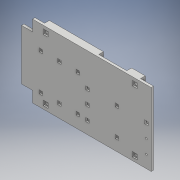
# Autodesk Inventor part: foot_printed
Saved by Autodesk Inventor 2018 (Build 220112000, 112)
## iProperties
Created: 2020-01-31
Part Number: foot_printed
Material: Generic
Document SubType Name: Modeling
Designer: bitbots
Density: 1 g/cm^3
Appearance: Default
Author: bitbots
Autodesk Inventor part; units mm, degrees
ref_plane "YZ Plane" through (0, 0, 0) normal (1, 0, 0) x (0, 1, 0)
ref_plane "XZ Plane" through (0, 0, 0) normal (0, 1, 0) x (-1, 0, 0)
ref_plane "XY Plane" through (0, 0, 0) normal (0, 0, 1) x (1, 0, 0)
sketch "Sketch1" plane through (0, 0, 0) normal (0, 1, 0) x (-1, 0, 0)
  line L0 (-65, 45) -> (65, 45) construction
  line L1 (65, 45) -> (65, -45) construction
  line L2 (65, -45) -> (-65, -45) construction
  line L3 (-65, -45) -> (-65, 45) construction
  line L4 (-65, 45) -> (65, -45) construction
  line L5 (65, 45) -> (-65, -45) construction
  circle A0 centre (65, 45) radius 2.1
  circle A1 centre (65, -45) radius 2.1
  circle A2 centre (-65, -45) radius 2.1
  circle A3 centre (-65, 45) radius 2.1
  line L6 (65, 45) -> (65, 19) construction
  line L7 (65, 19) -> (72, 19) construction
  line L8 (72, 19) -> (72, -34) construction
  line L9 (72, -34) -> (18, -34) construction
  line L10 (18, -34) -> (18, 19) construction
  line L11 (18, 19) -> (45, 19) construction
  line L12 (18, -34) -> (45, -34) construction
  circle A4 centre (45, -34) radius 1.35
  circle A5 centre (18, -34) radius 1.35
  circle A6 centre (18, 19) radius 1.35
  circle A7 centre (45, 19) radius 1.35
  circle A8 centre (72, -34) radius 1.35
  circle A9 centre (72, 19) radius 1.35
  line L13 (-65, -45) -> (-65, -35) construction
  line L14 (-65, -35) -> (-82, -35) construction
  circle A10 centre (-82, -35) radius 1.35
  line L15 (-82, -35) -> (-39, -35) construction
  line L16 (-39, -35) -> (4, -35) construction
  line L17 (4, -35) -> (4, -15) construction
  line L18 (4, -15) -> (4, 5) construction
  line L19 (4, 5) -> (-39, 5) construction
  line L20 (-39, 5) -> (-82, 5) construction
  circle A11 centre (-39, -35) radius 1.35
  circle A12 centre (4, -35) radius 1.35
  circle A13 centre (4, -15) radius 1.35
  circle A14 centre (4, 5) radius 1.35
  circle A15 centre (-39, 5) radius 1.35
  circle A16 centre (-82, 5) radius 1.35
  line L21 (-65, -45) -> (-65, -53) construction
  line L22 (-65, 45) -> (-65, 53) construction
  line L23 (65, -45) -> (65, -53) construction
  line L24 (65, 45) -> (70, 45) construction
  line L25 (65, 45) -> (65, 53) construction
  line L26 (-65, 45) -> (-70, 45) construction
  line L27 (-82, -35) -> (-89, -35) construction
  line L28 (-89, -35) -> (-89, -53)
  line L29 (-65, -53) -> (-89, -53)
  line L30 (-65, 53) -> (-89, 53)
  line L31 (-89, 53) -> (-89, -35)
  line L32 (-65, -53) -> (65, -53)
  line L33 (-65, 53) -> (65, 53)
  line L34 (65, -45) -> (100, -45) construction
  line L35 (100, -45) -> (100, -53)
  line L36 (100, -53) -> (65, -53)
  line L37 (65, 53) -> (100, 53)
  line L38 (100, 53) -> (100, -45)
  line L39 (-82, 5) -> (-82, -15) construction
  circle A17 centre (-82, -15) radius 1.35
  point P0 (0, 0)
  dimension "d0" = 130
  dimension "d1" = 90
  dimension "d2" = 4.2
  dimension "d3" = 4.2
  dimension "d4" = 4.2
  dimension "d5" = 4.2
  dimension "d6" = 26
  dimension "d7" = 7
  dimension "d8" = 53
  dimension "d9" = 54
  dimension "d10" = 53
  dimension "d11" = 27
  dimension "d12" = 27
  dimension "d13" = 2.7
  dimension "d14" = 2.7
  dimension "d15" = 2.7
  dimension "d16" = 2.7
  dimension "d17" = 2.7
  dimension "d18" = 2.7
  dimension "d19" = 10
  dimension "d20" = 17
  dimension "d21" = 2.7
  dimension "d22" = 43
  dimension "d23" = 43
  dimension "d24" = 20
  dimension "d26" = 20
  dimension "d27" = 43
  dimension "d28" = 43
  dimension "d29" = 2.7
  dimension "d30" = 2.7
  dimension "d31" = 2.7
  dimension "d32" = 2.7
  dimension "d33" = 2.7
  dimension "d34" = 2.7
  dimension "d35" = 8
  dimension "d36" = 8
  dimension "d38" = 8
  dimension "d40" = 5
  dimension "d41" = 8
  dimension "d42" = 5
  dimension "d43" = 7
  dimension "d44" = 35
  dimension "d54" = 20
  dimension "d55" = 2.7
  constraints: 80 end point, 18 centre point, 18 coincident, 14 perpendicular, 7 horizontal, 6 point on line, 6 vertical, 3 midpoint, 3 parallel
  measures "d0" distance of L1.end L2.end
  measures "d1" distance of L0.end L1.end
  measures "d2" diameter of A0
  measures "d3" diameter of A1
  measures "d4" diameter of A2
  measures "d5" diameter of A3
  measures "d6" distance of L6.start L6.end
  measures "d7" distance of L6.end L7.end
  measures "d8" distance of L7.end L8.end
  measures "d9" distance of L8.end L9.end
  measures "d10" distance of L9.end L10.end
  measures "d11" distance of L10.end L11.end
  measures "d12" distance of L9.end L12.end
  measures "d13" diameter of A4
  measures "d14" diameter of A5
  measures "d15" diameter of A6
  measures "d16" diameter of A7
  measures "d17" diameter of A8
  measures "d18" diameter of A9
  measures "d19" distance of L13.start L13.end
  measures "d20" distance of L13.end L14.end
  measures "d21" diameter of A10
  measures "d22" distance of L15.start L15.end
  measures "d23" distance of L15.end L16.end
  measures "d24" distance of L16.end L17.end
  measures "d26" distance of L17.end L18.end
  measures "d27" distance of L18.end L19.end
  measures "d28" distance of L19.end L20.end
  measures "d29" diameter of A11
  measures "d30" diameter of A12
  measures "d31" diameter of A13
  measures "d32" diameter of A14
  measures "d33" diameter of A15
  measures "d34" diameter of A16
  measures "d35" distance of L13.start L21.end
  measures "d36" distance of L22.start L22.end
  measures "d38" distance of L23.start L23.end
  measures "d40" distance of L6.start L24.end
  measures "d41" distance of L6.start L25.end
  measures "d42" distance of L22.start L26.end
  measures "d43" distance of L15.start L27.end
  measures "d44" distance of L23.start L34.end
  measures "d54" distance of L39.start L39.end
  measures "d55" diameter of A17
extrude "Extrusion1" add sketch "Sketch1" along normal blind 3.5
sketch "Sketch2" plane through (0, 3.5, 0) normal (0, 1, 0) x (1, 0, 0)
  circle A0 centre (65, -45) radius 2.1 construction
  circle A1 centre (65, 45) radius 2.1 construction
  circle A2 centre (-65, 45) radius 2.1 construction
  circle A3 centre (-65, -45) radius 2.1 construction
  circle A4 centre (82, -5) radius 1.35 construction
  circle A5 centre (39, -5) radius 1.35 construction
  circle A6 centre (-4, -5) radius 1.35 construction
  circle A7 centre (-4, 15) radius 1.35 construction
  circle A8 centre (-4, 35) radius 1.35 construction
  circle A9 centre (39, 35) radius 1.35 construction
  circle A10 centre (82, 35) radius 1.35 construction
  circle A11 centre (-72, -19) radius 1.35 construction
  circle A12 centre (-72, 34) radius 1.35 construction
  circle A13 centre (-45, -19) radius 1.35 construction
  circle A14 centre (-18, -19) radius 1.35 construction
  circle A15 centre (-18, 34) radius 1.35 construction
  circle A16 centre (-45, 34) radius 1.35 construction
  line L0 (89, 53) -> (-100, 53) construction
  line L1 (-100, 53) -> (-100, -53) construction
  line L2 (-100, -53) -> (89, -53) construction
  line L3 (89, -53) -> (89, 53) construction
  line L4 (65, -45) -> (65, -49.25) construction
  line L5 (65, -49.25) -> (60.75, -49.25)
  line L6 (60.75, -49.25) -> (60.75, -40.75)
  line L7 (60.75, -40.75) -> (65, -40.75)
  line L8 (65, -49.25) -> (70, -49.25)
  line L9 (65, -40.75) -> (70, -40.75)
  line L10 (89, -53) -> (-100, -53) construction
  line L11 (89, -53) -> (89, 53) construction
  line L12 (89, 0) -> (-100, 0) construction
  line L13 (0, 0) -> (0, 53) construction
  line L14 (89, 53) -> (-100, 53) construction
  line L15 (0, 0) -> (0, -53) construction
  line L16 (65, 49.25) -> (60.75, 49.25)
  line L17 (60.75, 49.25) -> (60.75, 40.75)
  line L18 (60.75, 40.75) -> (65, 40.75)
  line L19 (65, 49.25) -> (70, 49.25)
  line L20 (65, 40.75) -> (70, 40.75)
  line L21 (-65, -49.25) -> (-60.75, -49.25)
  line L22 (-60.75, -49.25) -> (-60.75, -40.75)
  line L23 (-60.75, -40.75) -> (-65, -40.75)
  line L24 (-65, -49.25) -> (-70, -49.25)
  line L25 (-65, -40.75) -> (-70, -40.75)
  line L26 (-60.75, 40.75) -> (-65, 40.75)
  line L27 (-65, 40.75) -> (-70, 40.75)
  line L28 (-65, 49.25) -> (-60.75, 49.25)
  line L29 (-65, 49.25) -> (-70, 49.25)
  line L30 (-60.75, 49.25) -> (-60.75, 40.75)
  line L31 (-70, -49.25) -> (-70, -53)
  line L32 (-70, -53) -> (70, -53) construction
  line L33 (70, -53) -> (70, -49.25)
  line L34 (70, 49.25) -> (70, 53)
  line L35 (70, 53) -> (-70, 53)
  line L36 (-70, 53) -> (-70, 49.25)
  line L37 (-70, -40.75) -> (-70, -37)
  circle A17 centre (-4, 35) radius 1.35 construction
  line L38 (-4, 35) -> (-11, 35) construction
  line L39 (-70, 40.75) -> (-70, 37)
  line L40 (-11, 35) -> (-11, 37)
  line L41 (-11, 37) -> (-70, 37)
  line L42 (-11, 35) -> (-11, -37)
  line L43 (-11, -37) -> (-70, -37)
  line L44 (-11, -37) -> (9, -37) construction
  line L45 (9, -37) -> (9, -53)
  line L46 (-100, -53) -> (89, -53) construction
  circle A18 centre (39, -5) radius 1.35 construction
  line L47 (39, -5) -> (39, -9) construction
  line L48 (39, -9) -> (9, -9) construction
  line L49 (9, -9) -> (9, -37)
  line L50 (9, -9) -> (-11, -9)
  line L51 (-4, 35) -> (-4, 39) construction
  line L52 (-4, 39) -> (-11, 39)
  line L53 (-11, 39) -> (-11, 37)
  line L54 (-4, 39) -> (70, 39)
  line L55 (70, 39) -> (70, 40.75)
  line L56 (70, -40.75) -> (70, -9)
  line L57 (-70, -53) -> (9, -53)
  line L58 (70, -53) -> (50, -53)
  line L59 (50, -53) -> (50, -9)
  line L60 (50, -9) -> (70, -9)
  dimension "d47" = 4.25
  dimension "d49" = 4.25
  dimension "d50" = 8.5
  dimension "d51" = 5
  dimension "d52" = 5
  dimension "d53" = 3.75
  dimension "d56" = 7
  dimension "d57" = 3.75
  dimension "d58" = 20
  dimension "d59" = 4
  dimension "d60" = 4
  dimension "d62" = 20
  constraints: 106 end point, 18 symmetric about line, 15 perpendicular, 12 point on line, 8 horizontal, 8 vertical, 2 midpoint, 1 collinear
  measures "d47" distance of L4.start L4.end
  measures "d49" distance of L4.end L5.end
  measures "d50" distance of L5.end L6.end
  measures "d51" distance of L4.end L8.end
  measures "d52" distance of L7.end L9.end
  measures "d53" distance of L25.end L37.end
  measures "d56" distance of L38.start L38.end
  measures "d57" distance of L27.end L39.end
  measures "d58" distance of L42.end L44.end
  measures "d59" distance of L47.start L47.end
  measures "d60" distance of L38.start L51.end
  measures "d62" distance of L32.end L58.end
extrude "Extrusion2" add sketch "Sketch2" along normal blind 7
sketch "Sketch3" plane through (0, 3.5, 0) normal (0, 1, 0) x (1, 0, 0)
  circle A0 centre (-45, 34) radius 1.35 construction
  circle A1 centre (-18, 34) radius 1.35 construction
  circle A2 centre (-18, -19) radius 1.35 construction
  circle A3 centre (-45, -19) radius 1.35 construction
  circle A4 centre (-72, 34) radius 1.35 construction
  circle A5 centre (-72, -19) radius 1.35 construction
  circle A6 centre (82, 35) radius 1.35 construction
  circle A7 centre (39, 35) radius 1.35 construction
  circle A8 centre (-4, 35) radius 1.35 construction
  circle A9 centre (-4, 15) radius 1.35 construction
  circle A10 centre (-4, -5) radius 1.35 construction
  circle A11 centre (39, -5) radius 1.35 construction
  circle A12 centre (82, -5) radius 1.35 construction
  circle A13 centre (82, 15) radius 1.35 construction
  circle A14 centre (-65, -45) radius 2.1 projected
  circle A15 centre (-65, 45) radius 2.1 projected
  circle A16 centre (65, 45) radius 2.1 projected
  circle A17 centre (65, -45) radius 2.1 projected
  line L0 (-70, -53) -> (-70, -49.25) projected
  line L1 (-70, -49.25) -> (-60.75, -49.25) projected
  line L2 (-60.75, -49.25) -> (-60.75, -40.75) projected
  line L3 (-60.75, -40.75) -> (-70, -40.75) projected
  line L4 (-70, -40.75) -> (-70, -37) projected
  line L5 (-70, -37) -> (-11, -37) construction
  line L6 (-11, -37) -> (-11, -9) construction
  line L7 (-11, -9) -> (9, -9) construction
  line L8 (9, -9) -> (9, -53) construction
  line L9 (9, -53) -> (50, -53) construction
  line L10 (50, -53) -> (50, -9) construction
  line L11 (50, -9) -> (70, -9) construction
  line L12 (70, -9) -> (70, -40.75) construction
  line L13 (70, -40.75) -> (60.75, -40.75) projected
  line L14 (60.75, -40.75) -> (60.75, -49.25) projected
  line L15 (60.75, -49.25) -> (70, -49.25) projected
  line L16 (70, -49.25) -> (70, -53) construction
  line L17 (70, -53) -> (89, -53) construction
  line L18 (89, -53) -> (89, 53) construction
  line L19 (89, 53) -> (70, 53) construction
  line L20 (70, 53) -> (70, 49.25) projected
  line L21 (70, 49.25) -> (60.75, 49.25) projected
  line L22 (60.75, 49.25) -> (60.75, 40.75) projected
  line L23 (60.75, 40.75) -> (70, 40.75) projected
  line L24 (70, 40.75) -> (70, 39) projected
  line L25 (70, 39) -> (-11, 39) construction
  line L26 (-11, 39) -> (-11, 37) construction
  line L27 (-11, 37) -> (-70, 37) construction
  line L28 (-70, 37) -> (-70, 40.75) construction
  line L29 (-70, 40.75) -> (-60.75, 40.75) projected
  line L30 (-60.75, 40.75) -> (-60.75, 49.25) projected
  line L31 (-60.75, 49.25) -> (-70, 49.25) projected
  line L32 (-70, 49.25) -> (-70, 53) construction
  line L33 (-70, 53) -> (-100, 53) construction
  line L34 (-100, 53) -> (-100, -53) construction
  line L35 (-100, -53) -> (-70, -53) construction
  line L36 (70, -49.25) -> (70, -40.75)
  line L37 (60.75, 49.25) -> (70, 49.25) projected
  line L38 (70, 40.75) -> (70, 49.25)
  line L39 (-70, 49.25) -> (-70, 40.75)
  line L40 (-70, -49.25) -> (-70, -40.75)
  point P0 (0, 0)
  constraints: 8 end point, 4 vertical
extrude "Extrusion3" add sketch "Sketch3" along normal blind 2
sketch "Sketch4" plane through (0, 10.5, 0) normal (0, 1, 0) x (1, 0, 0)
  circle A0 centre (65, -45) radius 2.1 projected
  line L0 (60.75, -40.75) -> (70, -40.75) projected
  line L1 (60.75, -49.25) -> (60.75, -40.75) projected
  line L2 (70, -49.25) -> (60.75, -49.25) projected
  line L3 (70, -49.25) -> (70, -40.75) projected
  circle A1 centre (65, 45) radius 2.1 projected
  line L4 (60.75, 49.25) -> (70, 49.25) projected
  line L5 (60.75, 40.75) -> (60.75, 49.25) projected
  line L6 (70, 40.75) -> (60.75, 40.75) projected
  line L7 (70, 40.75) -> (70, 49.25) projected
  circle A2 centre (-65, -45) radius 2.1 projected
  line L8 (-60.75, -49.25) -> (-70, -49.25) projected
  line L9 (-60.75, -40.75) -> (-60.75, -49.25) projected
  line L10 (-70, -40.75) -> (-60.75, -40.75) projected
  line L11 (-70, -40.75) -> (-70, -49.25) projected
  circle A3 centre (-65, 45) radius 2.1 projected
  line L12 (-60.75, 40.75) -> (-70, 40.75) projected
  line L13 (-60.75, 49.25) -> (-60.75, 40.75) projected
  line L14 (-70, 49.25) -> (-60.75, 49.25) projected
  line L15 (-70, 49.25) -> (-70, 40.75) projected
  point P0 (0, 0)
extrude "Extrusion4" add sketch "Sketch4" against normal blind 2
sketch "Sketch5" plane through (0, 3.5, 0) normal (0, 1, 0) x (1, 0, 0)
  circle A0 centre (-72, -19) radius 1.35 projected
  circle A1 centre (-45, -19) radius 1.35 projected
  circle A2 centre (-18, -19) radius 1.35 projected
  circle A3 centre (-18, 34) radius 1.35 projected
  circle A4 centre (-45, 34) radius 1.35 projected
  circle A5 centre (-72, 34) radius 1.35 projected
  circle A6 centre (-72, -19) radius 2.5
  circle A7 centre (-45, -19) radius 2.5
  circle A8 centre (-18, -19) radius 2.5
  circle A9 centre (-18, 34) radius 2.5
  circle A10 centre (-45, 34) radius 2.5
  circle A11 centre (-72, 34) radius 2.5
  point P0 (0, 0)
  dimension "d69" = 5
  dimension "d70" = 5
  dimension "d71" = 5
  dimension "d72" = 5
  dimension "d73" = 5
  dimension "d74" = 5
  constraints: 6 centre point, 6 coincident
  measures "d69" diameter of A6
  measures "d70" diameter of A7
  measures "d71" diameter of A8
  measures "d72" diameter of A9
  measures "d73" diameter of A10
  measures "d74" diameter of A11
extrude "Extrusion5" add sketch "Sketch5" along normal blind 2
sketch "Sketch6" plane through (0, 3.5, 0) normal (0, 1, 0) x (1, 0, 0)
  circle A0 centre (-45, 34) radius 2.5 construction
  circle A1 centre (-18, -19) radius 2.5 construction
  circle A2 centre (-72, -19) radius 2.5 construction
  circle A3 centre (-45, -19) radius 2.5 construction
  circle A4 centre (-18, 34) radius 2.5 construction
  circle A5 centre (-72, 34) radius 2.5 construction
  line L0 (70, 53) -> (70, 39) construction
  line L1 (70, 39) -> (-11, 39) construction
  line L2 (-11, 39) -> (-11, 37) construction
  line L3 (-11, 37) -> (-70, 37) construction
  line L4 (-70, 37) -> (-70, 53) construction
  line L5 (-70, 53) -> (-100, 53) construction
  line L6 (-100, 53) -> (-100, -53) construction
  line L7 (-100, -53) -> (-70, -53) construction
  line L8 (-70, -53) -> (-70, -37) construction
  line L9 (-70, -37) -> (-11, -37) construction
  line L10 (-11, -37) -> (-11, -9) construction
  line L11 (-11, -9) -> (9, -9) construction
  line L12 (9, -9) -> (9, -53) construction
  line L13 (9, -53) -> (50, -53) construction
  line L14 (50, -53) -> (50, -9) construction
  line L15 (50, -9) -> (70, -9) construction
  line L16 (70, -9) -> (70, -53) construction
  line L17 (70, -53) -> (89, -53) construction
  line L18 (89, -53) -> (89, 53) construction
  line L19 (89, 53) -> (70, 53) construction
  circle A6 centre (82, 35) radius 1.35 construction
  circle A7 centre (39, 35) radius 1.35 construction
  circle A8 centre (-4, 35) radius 1.35 construction
  circle A9 centre (-4, 15) radius 1.35 construction
  circle A10 centre (-4, -5) radius 1.35 construction
  circle A11 centre (39, -5) radius 1.35 construction
  circle A12 centre (82, -5) radius 1.35 construction
  circle A13 centre (82, 15) radius 1.35 construction
  line L20 (-100, 53) -> (-100, 37)
  line L21 (-100, 53) -> (-100, -53) projected
  line L22 (-100, 37) -> (-84, 37)
  line L23 (-84, 37) -> (-84, 53)
  line L24 (-100, 53) -> (89, 53) projected
  line L25 (-84, 53) -> (-100, 53)
  line L26 (-100, -53) -> (-100, -37)
  line L27 (-100, -37) -> (-84, -37)
  line L28 (-84, -53) -> (-84, -37)
  line L29 (-100, -53) -> (-84, -53)
  line L30 (89, -53) -> (-100, -53) projected
  point P0 (0, 0)
  dimension "d77" = 16
  dimension "d78" = 16
  dimension "d79" = 16
  constraints: 16 end point, 4 perpendicular, 4 point on line, 1 collinear, 1 horizontal
  measures "d77" distance of L20.end L22.end
  measures "d78" distance of L6.end L26.end
  measures "d79" distance of L26.end L27.end
extrude "Extrusion6" cut sketch "Sketch6" against normal through all
sketch "Sketch7" plane through (0, 0, 0) normal (0, -1, 0) x (1, 0, 0)
  line L0 (-84, -37) -> (-84, -53) construction
  line L1 (-84, -53) -> (89, -53) construction
  line L2 (89, -53) -> (89, 53) construction
  line L3 (89, 53) -> (-84, 53) construction
  line L4 (-84, 53) -> (-84, 37) construction
  line L5 (-84, 37) -> (-100, 37) construction
  line L6 (-100, 37) -> (-100, -37) construction
  line L7 (-100, -37) -> (-84, -37) construction
  circle A0 centre (65, 45) radius 2.1 construction
  circle A1 centre (65, -45) radius 2.1 construction
  circle A2 centre (-65, -45) radius 2.1 construction
  circle A3 centre (-65, 45) radius 2.1 construction
  circle A4 centre (82, -15) radius 1.35 construction
  circle A5 centre (82, 5) radius 1.35 construction
  circle A6 centre (39, 5) radius 1.35 construction
  circle A7 centre (-4, 5) radius 1.35 construction
  circle A8 centre (-4, -15) radius 1.35 construction
  circle A9 centre (-4, -35) radius 1.35 construction
  circle A10 centre (39, -35) radius 1.35 construction
  circle A11 centre (82, -35) radius 1.35 construction
  circle A12 centre (-72, 19) radius 1.35 construction
  circle A13 centre (-72, -34) radius 1.35 construction
  circle A14 centre (-45, 19) radius 1.35 construction
  circle A15 centre (-18, 19) radius 1.35 construction
  circle A16 centre (-18, -34) radius 1.35 construction
  circle A17 centre (-45, -34) radius 1.35 construction
  line L8 (-61.5, -48.5) -> (-68.5, -48.5)
  line L9 (-68.5, -48.5) -> (-68.5, -41.5)
  line L10 (-68.5, -41.5) -> (-61.5, -41.5)
  line L11 (-61.5, -41.5) -> (-61.5, -48.5)
  line L12 (-61.5, -48.5) -> (-68.5, -41.5) construction
  line L13 (-68.5, -48.5) -> (-61.5, -41.5) construction
  line L14 (-61.5, 48.5) -> (-68.5, 48.5)
  line L15 (-68.5, 48.5) -> (-68.5, 41.5)
  line L16 (-68.5, 41.5) -> (-61.5, 41.5)
  line L17 (-61.5, 41.5) -> (-61.5, 48.5)
  circle A18 centre (-65, 45) radius 2.1 projected
  line L18 (-61.5, 48.5) -> (-68.5, 41.5) construction
  line L19 (-68.5, 48.5) -> (-61.5, 41.5) construction
  line L20 (68.5, 48.5) -> (61.5, 48.5)
  line L21 (61.5, 48.5) -> (61.5, 41.5)
  line L22 (61.5, 41.5) -> (68.5, 41.5)
  line L23 (68.5, 41.5) -> (68.5, 48.5)
  line L24 (68.5, 48.5) -> (61.5, 41.5) construction
  line L25 (61.5, 48.5) -> (68.5, 41.5) construction
  line L26 (68.5, -48.5) -> (61.5, -48.5)
  line L27 (61.5, -48.5) -> (61.5, -41.5)
  line L28 (61.5, -41.5) -> (68.5, -41.5)
  line L29 (68.5, -41.5) -> (68.5, -48.5)
  line L30 (68.5, -48.5) -> (61.5, -41.5) construction
  line L31 (61.5, -48.5) -> (68.5, -41.5) construction
  line L32 (-69.5, -36.5) -> (-74.5, -36.5)
  line L33 (-74.5, -36.5) -> (-74.5, -31.5)
  line L34 (-74.5, -31.5) -> (-69.5, -31.5)
  line L35 (-69.5, -31.5) -> (-69.5, -36.5)
  line L36 (-69.5, -36.5) -> (-74.5, -31.5) construction
  line L37 (-74.5, -36.5) -> (-69.5, -31.5) construction
  line L38 (-69.5, 16.5) -> (-74.5, 16.5)
  line L39 (-74.5, 16.5) -> (-74.5, 21.5)
  line L40 (-74.5, 21.5) -> (-69.5, 21.5)
  line L41 (-69.5, 21.5) -> (-69.5, 16.5)
  line L42 (-69.5, 16.5) -> (-74.5, 21.5) construction
  line L43 (-74.5, 16.5) -> (-69.5, 21.5) construction
  line L44 (-42.5, -36.5) -> (-47.5, -36.5)
  line L45 (-47.5, -36.5) -> (-47.5, -31.5)
  line L46 (-47.5, -31.5) -> (-42.5, -31.5)
  line L47 (-42.5, -31.5) -> (-42.5, -36.5)
  line L48 (-42.5, -36.5) -> (-47.5, -31.5) construction
  line L49 (-47.5, -36.5) -> (-42.5, -31.5) construction
  line L50 (-15.5, -31.5) -> (-20.5, -31.5)
  line L51 (-20.5, -31.5) -> (-20.5, -36.5)
  line L52 (-20.5, -36.5) -> (-15.5, -36.5)
  line L53 (-15.5, -36.5) -> (-15.5, -31.5)
  line L54 (-15.5, -31.5) -> (-20.5, -36.5) construction
  line L55 (-20.5, -31.5) -> (-15.5, -36.5) construction
  line L56 (-42.5, 21.5) -> (-47.5, 21.5)
  line L57 (-47.5, 21.5) -> (-47.5, 16.5)
  line L58 (-47.5, 16.5) -> (-42.5, 16.5)
  line L59 (-42.5, 16.5) -> (-42.5, 21.5)
  line L60 (-42.5, 21.5) -> (-47.5, 16.5) construction
  line L61 (-47.5, 21.5) -> (-42.5, 16.5) construction
  line L62 (-20.5, 16.5) -> (-15.5, 16.5)
  line L63 (-15.5, 16.5) -> (-15.5, 21.5)
  line L64 (-15.5, 21.5) -> (-20.5, 21.5)
  line L65 (-20.5, 21.5) -> (-20.5, 16.5)
  circle A19 centre (-18, 19) radius 1.35 projected
  line L66 (-20.5, 16.5) -> (-15.5, 21.5) construction
  line L67 (-15.5, 16.5) -> (-20.5, 21.5) construction
  line L68 (-1.5, -32.5) -> (-6.5, -32.5)
  line L69 (-6.5, -32.5) -> (-6.5, -37.5)
  line L70 (-6.5, -37.5) -> (-1.5, -37.5)
  line L71 (-1.5, -37.5) -> (-1.5, -32.5)
  line L72 (-1.5, -32.5) -> (-6.5, -37.5) construction
  line L73 (-6.5, -32.5) -> (-1.5, -37.5) construction
  line L74 (-1.5, -12.5) -> (-6.5, -12.5)
  line L75 (-6.5, -12.5) -> (-6.5, -17.5)
  line L76 (-6.5, -17.5) -> (-1.5, -17.5)
  line L77 (-1.5, -17.5) -> (-1.5, -12.5)
  circle A20 centre (-4, -15) radius 1.35 projected
  line L78 (-1.5, -12.5) -> (-6.5, -17.5) construction
  line L79 (-6.5, -12.5) -> (-1.5, -17.5) construction
  line L80 (-6.5, 7.5) -> (-1.5, 7.5)
  line L81 (-1.5, 7.5) -> (-1.5, 2.5)
  line L82 (-1.5, 2.5) -> (-6.5, 2.5)
  line L83 (-6.5, 2.5) -> (-6.5, 7.5)
  line L84 (-6.5, 7.5) -> (-1.5, 2.5) construction
  line L85 (-1.5, 7.5) -> (-6.5, 2.5) construction
  line L86 (41.5, -37.5) -> (36.5, -37.5)
  line L87 (36.5, -37.5) -> (36.5, -32.5)
  line L88 (36.5, -32.5) -> (41.5, -32.5)
  line L89 (41.5, -32.5) -> (41.5, -37.5)
  line L90 (41.5, -37.5) -> (36.5, -32.5) construction
  line L91 (36.5, -37.5) -> (41.5, -32.5) construction
  line L92 (36.5, 2.5) -> (41.5, 2.5)
  line L93 (41.5, 2.5) -> (41.5, 7.5)
  line L94 (41.5, 7.5) -> (36.5, 7.5)
  line L95 (36.5, 7.5) -> (36.5, 2.5)
  circle A21 centre (39, 5) radius 1.35 projected
  line L96 (36.5, 2.5) -> (41.5, 7.5) construction
  line L97 (41.5, 2.5) -> (36.5, 7.5) construction
  line L98 (84.5, -37.5) -> (79.5, -37.5)
  line L99 (79.5, -37.5) -> (79.5, -32.5)
  line L100 (79.5, -32.5) -> (84.5, -32.5)
  line L101 (84.5, -32.5) -> (84.5, -37.5)
  circle A22 centre (82, -35) radius 1.35 projected
  line L102 (84.5, -37.5) -> (79.5, -32.5) construction
  line L103 (79.5, -37.5) -> (84.5, -32.5) construction
  line L104 (84.5, -17.5) -> (79.5, -17.5)
  line L105 (79.5, -17.5) -> (79.5, -12.5)
  line L106 (79.5, -12.5) -> (84.5, -12.5)
  line L107 (84.5, -12.5) -> (84.5, -17.5)
  circle A23 centre (82, -15) radius 1.35 projected
  line L108 (84.5, -17.5) -> (79.5, -12.5) construction
  line L109 (79.5, -17.5) -> (84.5, -12.5) construction
  line L110 (84.5, 2.5) -> (79.5, 2.5)
  line L111 (79.5, 2.5) -> (79.5, 7.5)
  line L112 (79.5, 7.5) -> (84.5, 7.5)
  line L113 (84.5, 7.5) -> (84.5, 2.5)
  line L114 (84.5, 2.5) -> (79.5, 7.5) construction
  line L115 (79.5, 2.5) -> (84.5, 7.5) construction
  point P0 (0, 0)
  dimension "d82" = 7
  dimension "d83" = 7
  dimension "d84" = 7
  dimension "d85" = 7
  dimension "d86" = 7
  dimension "d87" = 7
  dimension "d88" = 7
  dimension "d89" = 7
  dimension "d90" = 5
  dimension "d91" = 5
  dimension "d92" = 5
  dimension "d93" = 5
  dimension "d94" = 5
  dimension "d95" = 5
  dimension "d96" = 5
  dimension "d97" = 5
  dimension "d98" = 5
  dimension "d99" = 5
  dimension "d100" = 5
  dimension "d101" = 5
  dimension "d102" = 5
  dimension "d103" = 5
  dimension "d104" = 5
  dimension "d105" = 5
  dimension "d106" = 5
  dimension "d107" = 5
  dimension "d108" = 5
  dimension "d109" = 5
  dimension "d110" = 5
  dimension "d111" = 5
  dimension "d112" = 5
  dimension "d113" = 5
  dimension "d114" = 5
  dimension "d115" = 5
  dimension "d116" = 5
  dimension "d117" = 5
  constraints: 216 end point, 36 midpoint, 36 parallel, 18 horizontal, 18 perpendicular
  measures "d82" distance of L9.end L10.end
  measures "d83" distance of L8.end L9.end
  measures "d84" distance of L16.end L15.end
  measures "d85" distance of L15.end L14.end
  measures "d86" distance of L22.end L21.end
  measures "d87" distance of L21.end L20.end
  measures "d88" distance of L27.end L28.end
  measures "d89" distance of L26.end L27.end
  measures "d90" distance of L33.end L34.end
  measures "d91" distance of L32.end L33.end
  measures "d92" distance of L39.end L40.end
  measures "d93" distance of L38.end L39.end
  measures "d94" distance of L45.end L46.end
  measures "d95" distance of L44.end L45.end
  measures "d96" distance of L52.end L51.end
  measures "d97" distance of L51.end L50.end
  measures "d98" distance of L58.end L57.end
  measures "d99" distance of L57.end L56.end
  measures "d100" distance of L64.end L63.end
  measures "d101" distance of L63.end L62.end
  measures "d102" distance of L70.end L69.end
  measures "d103" distance of L69.end L68.end
  measures "d104" distance of L76.end L75.end
  measures "d105" distance of L75.end L74.end
  measures "d106" distance of L81.end L82.end
  measures "d107" distance of L80.end L81.end
  measures "d108" distance of L87.end L88.end
  measures "d109" distance of L86.end L87.end
  measures "d110" distance of L94.end L93.end
  measures "d111" distance of L93.end L92.end
  measures "d112" distance of L99.end L100.end
  measures "d113" distance of L98.end L99.end
  measures "d114" distance of L105.end L106.end
  measures "d115" distance of L104.end L105.end
  measures "d116" distance of L111.end L112.end
  measures "d117" distance of L110.end L111.end
extrude "Extrusion7" cut sketch "Sketch7" against normal blind 2 contours L8 L9 L10 L11 | L17 L16 L15 L14 | L23 L22 L21 L20 | L26 L27 L28 L29 | L32 L33 L34 L35 | L38 L39 L40 L41 | L44 L45 L46 L47 | L53 L52 L51 L50 | L59 L58 L57 L56 | L65 L64 L63 L62 | L71 L70 L69 L68 | L77 L76 L75 L74 | L80 L81 L82 L83 | L86 L87 L88 L89 | L95 L94 L93 L92 | A22 | A23 | L110 L111 L112 L113
chamfer "Chamfer1" distance 2 angle 45 6 edges at (-47.5, 3.5, 19) (-20.5, 3.5, 19) (-47.5, 3.5, -34) (-20.5, 3.5, -34) (-74.5, 3.5, 19) (-74.5, 3.5, -34)
equation "\"d3\" = d2"
equation "\"d4\" = d2"
equation "\"d5\" = d2"
equation "\"d22\" = d23"
equation "\"d27\" = d23"
equation "\"d28\" = d23"
equation "\"d49\" = d47"
equation "\"d50\" = 2 * d47"
body "Solid1"
